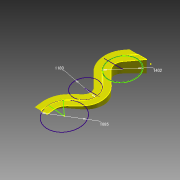
# Autodesk Inventor part: Down Hill_赤2
Saved by Autodesk Inventor 2015 (Build 190159000, 159)
## iProperties
Created: 2015-09-14
Part Number: Down Hill_赤2
Material: 一般
Document SubType Name: Modeling
Designer: nobuhiro
Density: 1 g/cm^3
Appearance: 滑らか - 黄
Author: nobuhiro
Autodesk Inventor part; units mm, degrees
ref_plane "YZ Plane" through (0, 0, 0) normal (1, 0, 0) x (0, 1, 0)
ref_plane "XZ Plane" through (0, 0, 0) normal (0, 1, 0) x (-1, 0, 0)
ref_plane "XY Plane" through (0, 0, 0) normal (0, 0, 1) x (1, 0, 0)
sketch "スケッチ1" plane through (0, 0, 0) normal (0, 0, 1) x (1, 0, 0)
  line L0 (1130.627776, 0) -> (1301.813888, -171.186112)
  line L1 (282.099639, 0) -> (877.549819, -595.450181)
  line L2 (1130.627776, 0) -> (282.099639, 0)
  circle A0 centre (594, -879) radius 1001 construction
  arc A1 (1296.712925, -1591.878353) -> (1296.712925, -1591.878353) centre (389.934597, -671.982591) ccw
  line L3 (1296.712925, -1591.878353) -> (686.416835, -2193.471806)
  circle A2 centre (890, -2400) radius 290 construction
  line L4 (713.355666, -2629.992999) -> (1149.394967, -2964.889592)
  line L5 (1595, -4169) -> (1595, -3869)
  circle A3 centre (455, -3869) radius 1140 construction
  arc A4 (875.506376, -1164.578641) -> (877.549819, -595.450181) centre (594, -879) ccw construction
  circle A5 centre (890, -2400) radius 890 construction
  circle A6 centre (455, -3869) radius 540 construction
  line L6 (783.923932, -3440.737175) -> (347.884631, -3105.840582)
  line L7 (265.210287, -1766.172094) -> (875.506376, -1164.578641)
  line L8 (995, -3869) -> (995, -4169)
  line L9 (995, -4169) -> (1595, -4169)
  arc A7 (1296.712925, -1591.878353) -> (1301.813888, -171.186112) centre (594, -879) ccw
  arc A8 (265.210287, -1766.172094) -> (347.884631, -3105.840582) centre (890, -2400) ccw
  arc A9 (686.416835, -2193.471806) -> (713.355666, -2629.992999) centre (890, -2400) ccw
  arc A10 (875.506376, -1164.578641) -> (877.549819, -595.450181) centre (594, -879) ccw
  arc A11 (995, -3869) -> (783.923932, -3440.737175) centre (455, -3869) ccw
  arc A12 (1595, -3869) -> (1149.394967, -2964.889592) centre (455, -3869) ccw
  line L10 (0, -4169) -> (1595, -4169) construction
  line L11 (1595, -4169) -> (1595, -4131.300846) construction
  line L12 (0, -4169) -> (0, 0) construction
  line L13 (0, 0) -> (1595, 0) construction
  line L14 (-1130.627776, 0) -> (-1301.813888, -171.186112)
  line L15 (-282.099639, 0) -> (-877.549819, -595.450181)
  line L16 (-1130.627776, 0) -> (-282.099639, 0)
  arc A13 (-1296.712925, -1591.878353) -> (-1296.712925, -1591.878353) centre (-389.934597, -671.982591) ccw
  line L17 (-1296.712925, -1591.878353) -> (-686.416835, -2193.471806)
  line L18 (-713.355666, -2629.992999) -> (-1149.394967, -2964.889592)
  line L19 (-1595, -4169) -> (-1595, -3869)
  line L20 (-783.923932, -3440.737175) -> (-347.884631, -3105.840582)
  line L21 (-265.210287, -1766.172094) -> (-875.506376, -1164.578641)
  line L22 (-995, -3869) -> (-995, -4169)
  line L23 (-995, -4169) -> (-1595, -4169)
  arc A14 (-1301.813888, -171.186112) -> (-1296.712925, -1591.878353) centre (-594, -879) ccw
  arc A15 (-347.884631, -3105.840582) -> (-265.210287, -1766.172094) centre (-890, -2400) ccw
  arc A16 (-713.355666, -2629.992999) -> (-686.416835, -2193.471806) centre (-890, -2400) ccw
  arc A17 (-877.549819, -595.450181) -> (-875.506376, -1164.578641) centre (-594, -879) ccw
  arc A18 (-783.923932, -3440.737175) -> (-995, -3869) centre (-455, -3869) ccw
  arc A19 (-1149.394967, -2964.889592) -> (-1595, -3869) centre (-455, -3869) ccw
  line L24 (0, -4169) -> (-1595, -4169) construction
  line L25 (-1595, -4169) -> (-1595, -4131.300846) construction
  line L26 (1595, -4169) -> (1595, 0) construction
  arc A20 (1120.235186, -2943.223489) -> (532.764288, -2869.555797) centre (890, -2400) ccw
  arc A21 (1086.10965, -1378.228497) -> (1089.681854, -383.318146) centre (594, -879) ccw
  line L27 (332.920262, 373.443445) -> (1089.681854, -383.318146)
  line L28 (475.813561, -1979.82195) -> (1086.10965, -1378.228497)
  arc A22 (1295, -3933.855609) -> (965.120487, -3198.490239) centre (455, -3869) ccw
  line L29 (1295, -4169) -> (1295, -3933.855609)
  line L30 (965.120487, -3198.490239) -> (532.764288, -2869.555797)
  dimension "d1" = 1080
  dimension "d2" = 2280
  dimension "d3" = 580
  dimension "d4" = 1780
  dimension "d5" = 802
  dimension "d6" = 2002
  dimension "d16" = 45
  dimension "d19" = 1140
  dimension "d20" = 4169
  dimension "d21" = 0
  dimension "d22" = 600
  dimension "d35" = 3290
  dimension "d36" = 1769
  dimension "d37" = 300
  dimension "d39" = 300
  dimension "d41" = 1595
  dimension "d43" = 1001
  dimension "d55" = 1180
  dimension "d58" = 1402
  dimension "d59" = 300
  dimension "d60" = 1685
  dimension "d61" = 300
  constraints: 62 end point, 49 point on circle, 26 symmetric about line, 23 centre point, 20 tangent, 4 horizontal, 3 coincident, 3 parallel, 2 concentric, 2 perpendicular, 2 point on line, 1 collinear, 1 vertical, 7 other
  measures "d1" diameter of A6
  measures "d2" diameter of A3
  measures "d3" diameter of A2
  measures "d4" diameter of A5
  measures "d5" diameter of A4
  measures "d6" diameter of A0
  measures "d16" angle of L13 L1
  measures "d19" distance from line of A6.centre L11
  measures "d20" distance between parallel lines of L13 L10
  measures "d21" distance between parallel lines of L11 L5
  measures "d22" distance of L8.end L5.start
  measures "d35" distance from line of L10 A0.centre
  measures "d36" distance from line of L10 A5.centre
  measures "d37" distance from line of L10 A3.centre
  measures "d39" distance from line of L10 A6.centre
  measures "d41" distance between parallel lines of L12 L26
  measures "d43" distance from line of L26 A4.centre
  measures "d55" diameter of A20
  measures "d58" diameter of A21
  measures "d59" distance between parallel lines of L27 L1
  measures "d60" diameter of A22
  measures "d61" distance from line of L5.start L29
extrude "押し出し1" add sketch "スケッチ1" along normal blind 600 contours L16 L15 A17 A1 | A1 A17 L21 A15 A13 A14 L14 L16 | A13 A15 L20 A18 L22 L23 L19 A19 L18 A16 L17 | L21 A15 A1
sketch "スケッチ2" plane through (0, 0, 0) normal (1, 0, 0) x (0, 1, 0)
  line L0 (0, 0) -> (0, 600)
  line L1 (0, 600) -> (-4169, 0)
  line L2 (-4169, 0) -> (0, 0)
  dimension "d26" = 600
  dimension "d27" = 4169
  constraints: 6 end point, 1 perpendicular, 1 vertical
  measures "d26" distance of L0.start L0.end
  measures "d27" distance of L1.end L0.start
extrude "押し出し2" cut sketch "スケッチ2" along normal through all both and the other way through all keep common part
sketch "スケッチ3" plane through (-1130.627776, 0, 600) normal (0, -0.1424517, 0.9898018) x (1, 0, 0)
  line L0 (0, 0) -> (-171.186112, -172.949897)
  ellipse E0 centre (536.627776, -888.056617) end of major axis (536.627776, 123.257005) minor radius 1001 (-171.186112, -172.949897) -> (-166.085149, -1608.279982) ccw
  line L1 (-166.085149, -1608.279982) -> (444.210941, -2216.071844)
  ellipse E1 centre (240.627776, -2424.727964) end of major axis (240.627776, -2131.740002) minor radius 290 (417.27211, -2657.090654) -> (444.210941, -2216.071844) ccw
  line L2 (417.27211, -2657.090654) -> (-18.767191, -2995.437793)
  ellipse E2 centre (675.627776, -3908.863539) end of major axis (675.627776, -2757.117756) minor radius 1140 (-18.767191, -2995.437793) -> (-464.372224, -3908.863539) ccw
  line L3 (-464.372224, -3908.863539) -> (-464.372224, -4211.954534)
  line L4 (-464.372224, -4211.954534) -> (135.627776, -4211.954534)
  line L5 (135.627776, -4211.954534) -> (135.627776, -3908.863539)
  ellipse E3 centre (675.627776, -3908.863539) end of major axis (675.627776, -4454.427331) minor radius 540 (346.703844, -3476.188186) -> (135.627776, -3908.863539) ccw
  line L6 (346.703844, -3476.188186) -> (782.743145, -3137.841046)
  ellipse E4 centre (240.627776, -2424.727964) end of major axis (240.627776, -3323.897918) minor radius 890 (782.743145, -3137.841046) -> (865.417489, -1784.369528) ccw
  line L7 (865.417489, -1784.369528) -> (255.1214, -1176.577665)
  ellipse E5 centre (536.627776, -888.056617) end of major axis (536.627776, -1293.188248) minor radius 401 (253.077957, -601.585294) -> (255.1214, -1176.577665) ccw
  line L8 (253.077957, -601.585294) -> (848.528137, 0)
  line L9 (848.528137, 0) -> (0, 0)
  line L10 (32.459504, -374.518685) -> (119.54728, -286.533616)
  line L11 (119.54728, -286.533616) -> (161.757904, -286.533616)
  line L12 (161.757904, -286.533616) -> (49.432341, -400.016505)
  line L13 (52.928503, -1379.603638) -> (663.224592, -1987.395501)
  line L14 (607.085651, -2911.465345) -> (171.04635, -3249.812485)
  line L15 (-150.90584, -3908.863539) -> (-150.90584, -3925.420918)
  line L16 (-150.90584, -3925.420918) -> (-177.838608, -3925.420918)
  line L17 (-177.838608, -3925.420918) -> (-177.838608, -3908.863539)
  line L18 (156.890303, -3221.813494) -> (592.929604, -2883.466355)
  line L19 (646.403838, -2013.045871) -> (36.107748, -1405.254009)
  line L20 (-177.838608, -3925.420918) -> (-177.838608, -4211.954534)
  line L21 (-150.90584, -3925.420918) -> (-150.90584, -4211.954534)
  line L22 (119.54728, -286.533616) -> (403.158757, 0)
  line L23 (161.757904, -286.533616) -> (445.369381, 0)
  line L24 (135.627776, -4196.954534) -> (-464.372224, -4196.954534)
  circle A0 centre (536.627776, -888.056617) radius 687.533623
  circle A1 centre (536.627776, -888.056617) radius 714.466404
  circle A2 centre (536.627776, -888.056617) radius 702.533623
  line L25 (536.627776, -888.056617) -> (-165.905847, -888.056617)
  spline S0 degree 5 poles (49.432313, -400.016478) (6.077227, -443.818375) (-32.384649, -492.463466) (-65.245601, -545.209886) (-132.816663, -686.686848) (-159.115063, -842.537878) (-158.773953, -938.579626) (-131.367798, -1094.241054) (-62.788599, -1235.233354) (-29.550818, -1287.744456) (9.259286, -1336.113556) (52.928475, -1379.603666) knots 0 0 0 0 0 0 0.28340783 0.28340783 0.28340783 0.71658777 0.71658777 0.71658777 1 1 1 1 1 1
  spline S1 degree 5 poles (663.224587, -1987.395506) (689.075742, -2013.14062) (712.995547, -2040.825086) (734.798846, -2070.246947) (790.871239, -2159.036636) (827.290897, -2258.293566) (841.913972, -2325.841291) (852.274256, -2463.111073) (825.311564, -2598.10068) (802.618247, -2663.275174) (754.460895, -2757.168939) (688.062902, -2838.256606) (662.887271, -2864.702619) (635.825083, -2889.164768) (607.085644, -2911.465337) knots 0 0 0 0 0 0 0.17436211 0.17436211 0.17436211 0.50050025 0.50050025 0.50050025 0.826151 0.826151 0.826151 1 1 1 1 1 1
  spline S2 degree 5 poles (171.046331, -3249.81246) (111.042432, -3296.372766) (56.382455, -3349.819709) (8.104424, -3409.315106) (-74.022271, -3538.251051) (-125.0897, -3682.339847) (-142.300458, -3756.981031) (-150.905856, -3832.922299) (-150.905852, -3908.863539) knots 0 0 0 0 0 0 0.50002711 0.50002711 0.50002711 1 1 1 1 1 1
  spline S3 degree 5 poles (-177.8386, -3908.863539) (-177.838569, -3829.462861) (-168.853548, -3750.06212) (-150.883663, -3672.016939) (-97.718356, -3521.8667) (-12.219082, -3387.492156) (37.862436, -3325.6829) (94.589087, -3270.156386) (156.890287, -3221.813474) knots 0 0 0 0 0 0 0.50171698 0.50171698 0.50171698 1 1 1 1 1 1
  spline S4 degree 5 poles (592.929643, -2883.466405) (637.116056, -2849.179555) (677.147225, -2809.537849) (712.168719, -2765.225935) (786.283528, -2643.702753) (821.3073, -2504.348583) (826.632167, -2417.149407) (808.848433, -2274.604137) (750.159778, -2144.96338) (720.849211, -2096.723221) (686.010859, -2052.490454) (646.403872, -2013.045836) knots 0 0 0 0 0 0 0.28358577 0.28358577 0.28358577 0.71657004 0.71657004 0.71657004 1 1 1 1 1 1
  spline S5 degree 5 poles (36.107752, -1405.254005) (7.864752, -1377.12687) (-18.430404, -1347.043832) (-42.604908, -1315.192514) (-105.462623, -1219.337185) (-148.735449, -1112.473232) (-167.867897, -1039.634178) (-187.271249, -890.697388) (-168.925567, -741.626429) (-150.309509, -668.648054) (-107.794348, -561.468167) (-45.617295, -465.156101) (-21.667813, -433.127656) (4.41493, -402.852244) (32.459508, -374.518689) knots 0 0 0 0 0 0 0.17426528 0.17426528 0.17426528 0.49997454 0.49997454 0.49997454 0.82570808 0.82570808 0.82570808 1 1 1 1 1 1
  point P0 (1130.627776, -85.471008)
  dimension "d31" = 30
  dimension "d32" = 15
  dimension "d62" = 1428.93281
  dimension "d63" = 15
  constraints: 32 end point, 11 parallel, 6 point on line, 3 coincident, 2 centre point, 2 collinear, 2 perpendicular, 1 horizontal, 1 horizontal alignment, 1 vertical, 30 other
  measures "d31" distance between parallel lines of L12 L10
  measures "d32" distance between parallel lines of L4 L24
  measures "d62" diameter of A1
sketch "スケッチ3 outline for 押し出し3" plane through (-1130.627776, 0, 600) normal (0, -0.1424517, 0.9898018) x (1, 0, 0)
  line L0 (403.158757, 0) -> (119.54728, -286.533616)
  line L1 (119.54728, -286.533616) -> (32.459508, -374.518689)
  spline S0 degree 5 poles (36.107752, -1405.254005) (7.864752, -1377.12687) (-18.430404, -1347.043832) (-42.604908, -1315.192514) (-105.462623, -1219.337185) (-148.735449, -1112.473232) (-167.867897, -1039.634178) (-187.271249, -890.697388) (-168.925567, -741.626429) (-150.309509, -668.648054) (-107.794348, -561.468167) (-45.617295, -465.156101) (-21.667813, -433.127656) (4.41493, -402.852244) (32.459508, -374.518689) knots 0 0 0 0 0 0 0.17426528 0.17426528 0.17426528 0.49997454 0.49997454 0.49997454 0.82570808 0.82570808 0.82570808 1 1 1 1 1 1
  line L2 (36.107752, -1405.254005) -> (646.403838, -2013.045871)
  spline S1 degree 5 poles (592.929643, -2883.466405) (637.116056, -2849.179555) (677.147225, -2809.537849) (712.168719, -2765.225935) (786.283528, -2643.702753) (821.3073, -2504.348583) (826.632167, -2417.149407) (808.848433, -2274.604137) (750.159778, -2144.96338) (720.849211, -2096.723221) (686.010859, -2052.490454) (646.403838, -2013.045871) knots 0 0 0 0 0 0 0.28358577 0.28358577 0.28358577 0.71657004 0.71657004 0.71657004 1 1 1 1 1 1
  line L3 (592.929643, -2883.466405) -> (156.890303, -3221.813494)
  spline S2 degree 5 poles (-177.8386, -3908.863539) (-177.838569, -3829.462861) (-168.853548, -3750.06212) (-150.883663, -3672.016939) (-97.718356, -3521.8667) (-12.219082, -3387.492156) (37.862436, -3325.6829) (94.589087, -3270.156386) (156.890303, -3221.813494) knots 0 0 0 0 0 0 0.50171698 0.50171698 0.50171698 1 1 1 1 1 1
  line L4 (-177.8386, -3908.863539) -> (-177.838608, -3925.420918)
  line L5 (-177.838608, -3925.420918) -> (-177.838608, -4211.954534)
  line L6 (-177.838608, -4211.954534) -> (-150.90584, -4211.954534)
  line L7 (-150.90584, -4211.954534) -> (-150.90584, -3908.863539)
  spline S3 degree 5 poles (171.046331, -3249.81246) (111.042432, -3296.372766) (56.382455, -3349.819709) (8.104424, -3409.315106) (-74.022271, -3538.251051) (-125.0897, -3682.339847) (-142.300458, -3756.981031) (-150.905856, -3832.922299) (-150.90584, -3908.863539) knots 0 0 0 0 0 0 0.50002711 0.50002711 0.50002711 1 1 1 1 1 1
  line L8 (171.046331, -3249.81246) -> (607.085651, -2911.465345)
  spline S4 degree 5 poles (663.224587, -1987.395506) (689.075742, -2013.14062) (712.995547, -2040.825086) (734.798846, -2070.246947) (790.871239, -2159.036636) (827.290897, -2258.293566) (841.913972, -2325.841291) (852.274256, -2463.111073) (825.311564, -2598.10068) (802.618247, -2663.275174) (754.460895, -2757.168939) (688.062902, -2838.256606) (662.887271, -2864.702619) (635.825083, -2889.164768) (607.085651, -2911.465345) knots 0 0 0 0 0 0 0.17436211 0.17436211 0.17436211 0.50050025 0.50050025 0.50050025 0.826151 0.826151 0.826151 1 1 1 1 1 1
  line L9 (663.224587, -1987.395506) -> (52.928503, -1379.603638)
  spline S5 degree 5 poles (49.432313, -400.016478) (6.077227, -443.818375) (-32.384649, -492.463466) (-65.245601, -545.209886) (-132.816663, -686.686848) (-159.115063, -842.537878) (-158.773953, -938.579626) (-131.367798, -1094.241054) (-62.788599, -1235.233354) (-29.550818, -1287.744456) (9.259286, -1336.113556) (52.928503, -1379.603638) knots 0 0 0 0 0 0 0.28340783 0.28340783 0.28340783 0.71658777 0.71658777 0.71658777 1 1 1 1 1 1
  line L10 (49.432313, -400.016478) -> (161.757904, -286.533616)
  line L11 (161.757904, -286.533616) -> (445.369381, 0)
  line L12 (445.369381, 0) -> (403.158757, 0)
extrude "押し出し3" add sketch "スケッチ3 outline for 押し出し3" along normal blind 0.1
sketch "スケッチ5" plane through (0, 0, 0) normal (0, 0, 1) x (1, 0, 0)
  line L0 (-1308.466384, -3869.014245) -> (-1308.466384, -4169.014245)
  line L1 (-1308.466384, -4169.014245) -> (-1281.533616, -4169.014245)
  line L2 (-1281.533616, -4169.014245) -> (-1281.533616, -3869.014245)
  line L3 (-959.581426, -3216.684354) -> (-523.542125, -2881.78776)
  line L4 (-467.403184, -1967.141804) -> (-1077.699273, -1365.548351)
  line L5 (-1081.195435, -395.951285) -> (-685.258395, -0.014245)
  line L6 (-685.258395, -0.014245) -> (-727.469019, -0.014245)
  line L7 (-727.469019, -0.014245) -> (-1098.168272, -370.713498)
  line L8 (-1094.520028, -1390.937133) -> (-484.223938, -1992.530586)
  line L9 (-537.698172, -2854.07431) -> (-973.737473, -3188.970904)
  line L10 (-1081.195435, -395.951285) -> (-598.117629, -879.029091)
  line L11 (-598.117629, -879.029091) -> (-1077.699273, -1365.548351)
  line L12 (-598.117629, -879.029091) -> (-1281.52915, -881.482864)
  line L13 (-1281.52915, -881.482864) -> (-1308.461836, -881.579565)
  line L14 (-484.223938, -1992.530586) -> (-886.199659, -2400.321278)
  line L15 (-886.199659, -2400.321278) -> (-537.698172, -2854.07431)
  line L16 (-886.199659, -2400.321278) -> (-314.576724, -2435.597581)
  line L17 (-314.576724, -2435.597581) -> (-287.672956, -2437.257881)
  line L18 (-1281.533616, -3869.014245) -> (-458.564526, -3869.014245)
  line L19 (-458.564526, -3869.014245) -> (-959.581426, -3216.684354)
  line L20 (-458.564526, -3869.014245) -> (-1196.563908, -3505.279644)
  line L21 (-1196.563908, -3505.279644) -> (-1221.734569, -3492.873888)
  point P0 (0, 0)
  point P1 (-1294.995493, -881.531215)
  point P2 (-301.12484, -2436.427731)
  point P3 (-1209.149239, -3499.076766)
  point P4 (536.976093, 8076.719831)
  dimension "d44" = 669.93748
  dimension "d45" = 1732.58651
  dimension "d46" = 3287.48303
  constraints: 24 end point, 3 collinear, 3 midpoint, 1 horizontal, 20 other
  measures "d44" distance from line of L1 point (-1209.149, -3499.077)
  measures "d45" distance from line of L1 point (-301.125, -2436.428)
  measures "d46" distance from line of point (-1294.995, -881.531) L1
sketch "スケッチ6" plane through (0, 0, 0) normal (1, 0, 0) x (0, 1, 0)
  line L0 (-3869.014245, 43.274802) -> (-4169.014245, 0.09898)
  line L1 (-4169.014245, 0.09898) -> (-3869.014245, 43.274802)
  line L2 (-3869.014245, 43.274802) -> (-3216.684354, 137.157732)
  line L3 (-3216.684354, 137.157732) -> (-2881.78776, 185.35585)
  line L4 (-2881.78776, 185.35585) -> (-1967.141804, 316.991152)
  line L5 (-1967.141804, 316.991152) -> (-1365.548351, 403.572124)
  line L6 (-1365.548351, 403.572124) -> (-395.951285, 543.115957)
  line L7 (-395.951285, 543.115957) -> (-0.014245, 600.09898)
  line L8 (-0.014245, 600.09898) -> (-370.713498, 546.748164)
  line L9 (-370.713498, 546.748164) -> (-1390.937133, 399.918186)
  line L10 (-1390.937133, 399.918186) -> (-1992.530586, 313.337214)
  line L11 (-1992.530586, 313.337214) -> (-2854.07431, 189.344353)
  line L12 (-2854.07431, 189.344353) -> (-3188.970904, 141.146235)
  line L13 (-3188.970904, 141.146235) -> (-3869.014245, 43.274802)
  point P0 (0, 0)
  point P1 (-3499.076766, 96.515984)
  point P2 (-2436.427731, 249.451801)
  point P3 (-881.531215, 473.231582)
  dimension "d47" = 669.93748
  dimension "d48" = 1732.58651
  dimension "d49" = 3287.48303
  dimension "d50" = 96.417
  dimension "d51" = 249.35282
  dimension "d52" = 473.1326
  constraints: 3 point on line
  measures "d47" horizontal distance of point (-3499.077, 96.516) L0.end
  measures "d48" horizontal distance of L0.end point (-2436.428, 249.452)
  measures "d49" horizontal distance of L0.end point (-881.531, 473.232)
  measures "d50" vertical distance of point (-3499.077, 96.516) L0.end
  measures "d51" vertical distance of L0.end point (-2436.428, 249.452)
  measures "d52" vertical distance of L0.end point (-881.531, 473.232)
sketch "スケッチ7" plane through (-1130.627776, -0.014245, 600.09898) normal (0, -0.1424517, 0.9898018) x (1, 0, 0)
  line L0 (-177.838608, -3908.863539) -> (-177.838608, -4211.954534)
  line L1 (-177.838608, -4211.954534) -> (-150.90584, -4211.954534)
  line L2 (-150.90584, -4211.954534) -> (-150.90584, -3908.863539)
  line L3 (171.04635, -3249.812485) -> (607.085651, -2911.465345)
  line L4 (663.224592, -1987.395501) -> (52.928503, -1379.603638)
  line L5 (49.432341, -400.016505) -> (445.369381, 0)
  line L6 (445.369381, 0) -> (403.158757, 0)
  line L7 (403.158757, 0) -> (32.459504, -374.518685)
  line L8 (36.107748, -1405.254009) -> (646.403838, -2013.045871)
  line L9 (592.929604, -2883.466355) -> (156.890303, -3221.813494)
  line L10 (-150.90584, -3908.863539) -> (-150.90584, -4211.954534)
  line L11 (-150.90584, -4211.954534) -> (135.627776, -4211.954534)
  line L12 (135.627776, -4211.954534) -> (135.627776, -3908.863539)
  ellipse E0 centre (675.627776, -3908.863539) end of major axis (675.627776, -4454.427331) minor radius 540 (346.703844, -3476.188186) -> (135.627776, -3908.863539) ccw
  line L13 (346.703844, -3476.188186) -> (782.743145, -3137.841046)
  ellipse E1 centre (240.627776, -2424.727964) end of major axis (240.627776, -3323.897918) minor radius 890 (782.743145, -3137.841046) -> (865.417489, -1784.369528) ccw
  line L14 (865.417489, -1784.369528) -> (255.1214, -1176.577665)
  ellipse E2 centre (536.627776, -888.056617) end of major axis (536.627776, -1293.188248) minor radius 401 (253.077957, -601.585294) -> (255.1214, -1176.577665) ccw
  line L15 (253.077957, -601.585294) -> (848.528137, 0)
  line L16 (848.528137, 0) -> (445.369381, 0)
  line L17 (445.369381, 0) -> (49.432341, -400.016505)
  line L18 (52.928503, -1379.603638) -> (663.224592, -1987.395501)
  line L19 (607.085651, -2911.465345) -> (171.04635, -3249.812485)
  line L20 (536.627776, -888.056617) -> (-363.574656, -888.056617)
  line L21 (240.627776, -2424.727964) -> (865.417489, -2424.727964)
  circle A0 centre (675.627776, -3908.863539) radius 842.5
  circle A1 centre (240.627776, -2424.727964) radius 590
  circle A2 centre (536.627776, -888.056617) radius 701
  line L22 (675.627776, -3908.863539) -> (-164.372224, -3844.00793)
  line L23 (675.627776, -3908.863539) -> (52.620076, -3341.706016)
  circle A3 centre (536.627776, -888.056617) radius 714.466403
  circle A4 centre (536.627776, -888.056617) radius 687.533623
  point P0 (1130.627776, -85.471008)
  point P1 (-164.372224, -888.056617)
  point P2 (830.627776, -2424.727964)
  point P3 (-164.372224, -888.056617)
  point P4 (830.627776, -2424.727964)
  dimension "d56" = 1180
  dimension "d57" = 1402
  dimension "d54" = 1685
  constraints: 8 coincident, 8 end point, 3 centre point, 2 horizontal, 2 horizontal alignment, 2 point on circle, 2 point on line, 16 other
  measures "d54" diameter of A0
equation "\"d47\" = d44"
equation "\"d48\" = d45"
equation "\"d49\" = d46"
